Autodesk Fusion 360 part; units mm, degrees
(part 2 of 2)
  constraint concentric A5 A228
  constraint concentric A26 A229
  constraint concentric A24 A230
  constraint concentric A23 A231
  constraint concentric A22 A232
  constraint concentric A21 A233
  constraint concentric A20 A234
  constraint concentric A19 A235
  constraint concentric A18 A236
  constraint concentric A17 A237
  constraint concentric A16 A238
  constraint concentric A15 A239
  constraint concentric A14 A240
  constraint concentric A13 A241
  constraint tangent L211 A241
  constraint tangent A220 L212
  constraint tangent A222 L214
  constraint tangent A240 L232
  constraint tangent A235 L227
  constraint tangent A221 L213
  constraint tangent L212 A221
  constraint tangent A236 L228
  constraint tangent A223 L215
  constraint tangent A224 L216
  constraint tangent A225 L217
  constraint tangent A226 L218
  constraint tangent A239 L231
  constraint tangent A227 L219
  constraint tangent A231 L223
  constraint tangent L219 A228
  constraint tangent A229 L221
  constraint tangent L221 A230
  constraint tangent A234 L226
  constraint tangent A230 L222
  constraint tangent A232 L224
  constraint tangent A233 L225
  constraint tangent A237 L229
  constraint tangent A238 L230
  constraint concentric A220 A242
  constraint concentric A222 A243
  constraint concentric A224 A244
  constraint concentric A225 A245
  constraint concentric A227 A246
  constraint concentric A229 A247
  constraint concentric A230 A248
  constraint concentric A231 A249
  constraint concentric A233 A250
  constraint concentric A235 A251
  constraint concentric A238 A252
  constraint concentric A239 A253
  constraint concentric A240 A254
  constraint tangent A243 L234
  constraint tangent A245 L237
  constraint tangent A246 L239
  constraint tangent A247 L241
  constraint tangent L241 A248
  constraint tangent A253 L248
  constraint tangent A249 L243
  constraint tangent A250 L245
  constraint tangent A254 L249
  constraint tangent A252 L247
  constraint tangent A242 L250
  constraint tangent A243 L251
  constraint tangent A252 L252
  constraint coincident L220 L177.start
  constraint coincident L240 L177.end
  constraint coincident L221 L178.start
  constraint coincident L241 L178.end
  constraint tangent L252 A255
  constraint tangent A255 L253
  constraint tangent A251 L254
  constraint tangent L253 A256
  constraint tangent L254 A256
  constraint tangent L245 A257
  constraint tangent L246 A257
  constraint tangent L243 A258
  constraint tangent L244 A258
  constraint tangent L239 A259
  constraint tangent L240 A259
  constraint tangent L237 A260
  constraint tangent L238 A260
  constraint tangent L234 A261
  constraint tangent L235 A261
  constraint tangent L250 A262
  constraint tangent L251 A262
  constraint tangent L233 A263
  constraint tangent L249 A263
  constraint tangent L203 A264
  constraint tangent L203 A265
  constraint tangent L255 A266
  constraint tangent L255 A267
  measures "d1" diameter of A0
  measures "d2" diameter of A1
  measures "d3" diameter of A2
  measures "d4" diameter of A3
  measures "d5" diameter of A4
  measures "d9" diameter of A111
  measures "d12" diameter of A112
  measures "d396" diameter of A218
  measures "d397" diameter of A219
  measures "d418" radius of A255
  measures "d419" radius of A256
  measures "d420" radius of A257
  measures "d421" radius of A258
  measures "d422" radius of A259
  measures "d423" radius of A260
  measures "d424" radius of A261
  measures "d425" radius of A262
  measures "d426" radius of A263
extrude "Extrude1" add sketch "mriya-bumper-fdm" along normal blind 10.7 contours L177 L178 L211 A220 L212 A221 L213 A222 L214 A223 L215 A224 L216 A225 L217 A226 L218 A227 L219 A228 L220 L221 A230 L222 A231 L223 A232 L224 A233 L225 A234 L226 A235 L227 A236 L228 A237 L229 A238 L230 A239 L231 A240 L232 A241 L233 A242 A243 L234 L235 A244 L236 A245 L237 L238 A246 L239 L240 L241 A248 L242 A249 L243 L244 A250 L245 L246 A251 A252 L247 A253 L248 A254 L249 L250 L251 L252 A255 L253 L254 A256 A257 A258 A259 A260 A261 A262 A263 makes body 1
extrude "Extrude2" add sketch "mriya-bumper-fdm" along normal blind 17.3 contours L177 L178 L220 A229 L221 L240 A247 L241 bodies 1
extrude "Extrude3" add sketch "mriya-bumper-fdm" along normal blind 2 from surface at 1.9 contours A114 | A115 | A116 | A117 | L203 L211 A220 L212 A221 L213 A222 L214 A223 L215 A224 L216 A225 L217 A226 L218 A227 L219 A228 L220 A229 L221 A230 L222 A231 L223 A232 L224 A233 L225 A234 L226 A235 L227 A236 L228 A237 L229 A238 L230 A239 L231 A240 L232 A241 L255 A264 A265 A266 A267 | L203 L220 A264 A265 | L221 L255 A266 A267 bodies 1
extrude "Extrude6" add sketch "mriya-bumper-fdm" along normal blind 1.2 from surface at 14.3 contours L203 L220 A264 A265 bodies 1
extrude "Extrude12" add sketch "mriya-bumper-fdm" along normal blind 1.2 from surface at 7.7 contours L221 L255 A266 A267 bodies 1
sketch "power-switch" plane through (-4.28, 0, 0) normal (1, 0, 0) x (0, 1, 0)
  line L0 (25.7932, 5.6) -> (25.7932, 8.5)
  line L1 (35.9932, 5.6) -> (25.7932, 5.6)
  arc A0 (37.3932, 4.25) -> (37.7932, 4.65) centre (37.3932, 4.65) ccw
  arc A1 (24.3932, 9.85) -> (23.9932, 9.45) centre (24.3932, 9.45) ccw
  line L2 (23.9932, 4.65) -> (23.9932, 9.45)
  line L3 (25.7932, 8.5) -> (35.9932, 8.5)
  arc A2 (23.9932, 4.65) -> (24.3932, 4.25) centre (24.3932, 4.65) ccw
  line L4 (37.7932, 9.45) -> (37.7932, 4.65)
  line L5 (37.3932, 4.25) -> (24.3932, 4.25)
  line L6 (24.3932, 9.85) -> (37.3932, 9.85)
  line L7 (35.9932, 8.5) -> (35.9932, 5.6)
  arc A3 (37.7932, 9.45) -> (37.3932, 9.85) centre (37.3932, 9.45) ccw
  line L8 (1.9932, 0) -> (76.4932, 0)
  line L9 (76.4932, 0) -> (76.4932, 17.3)
  line L10 (76.4932, 17.3) -> (19.3932, 17.3)
  line L11 (19.3932, 17.3) -> (19.3932, 10.7)
  line L12 (19.3932, 10.7) -> (1.9932, 10.7)
  line L13 (1.9932, 10.7) -> (1.9932, 0)
  constraint perpendicular L0 L1
  constraint vertical L0
  constraint perpendicular L0 L3
  constraint vertical L7
  constraint tangent L6 A3
  constraint tangent L4 A3
  constraint tangent A0 L4
  constraint tangent A0 L5
  constraint tangent A2 L5
  constraint tangent L2 A2
  constraint tangent A1 L2
  constraint tangent A1 L6
extrude "Extrude8" cut sketch "power-switch" against normal blind 2.6 contours L0 L1 L3 L7 bodies 1
extrude "Extrude9" cut sketch "power-switch" against normal blind 1.2 contours A0 A1 L2 A2 L4 L5 L6 A3 bodies 1
chamfer "Chamfer13" distance 1.43 angle 40 8 edges at (-4.28, 30.8932, 4.25) (-4.28, 24.1104, 4.3672) (-4.28, 23.9932, 7.05) (-4.28, 24.1104, 9.7328) (-4.28, 30.8932, 9.85) (-4.28, 37.676, 9.7328) (-4.28, 37.7932, 7.05) (-4.28, 37.676, 4.3672) measured on face at (-4.28, 63.5932, 8.9167) measured on face at (-4.28, 63.5932, 8.9167) measured on face at (-4.28, 63.5932, 8.9167) measured on face at (-4.28, 63.5932, 8.9167) measured on face at (-4.28, 63.5932, 8.9167) measured on face at (-4.28, 63.5932, 8.9167) measured on face at (-4.28, 63.5932, 8.9167) measured on face at (-4.28, 63.5932, 8.9167) on bodies 1
sketch "usb-c" plane through (0, 80.8132, 0) normal (0, 1, 0) x (-1, 0, 0)
  line L0 (11.0002, 8.4) -> (11.0002, 13.2)
  line L1 (21.0002, 11.4) -> (21.0002, 10.2)
  line L2 (11.8003, 10.2) -> (11.8003, 11.4)
  arc A0 (11.4002, 13.6) -> (11.0002, 13.2) centre (11.4002, 13.2) ccw
  line L3 (11.4002, 13.6) -> (21.4002, 13.6)
  line L4 (21.8003, 13.2) -> (21.8003, 8.4)
  arc A1 (21.8003, 13.2) -> (21.4002, 13.6) centre (21.4002, 13.2) ccw
  arc A2 (21.4002, 8) -> (21.8002, 8.4) centre (21.4002, 8.4) ccw
  line L5 (13.0003, 12.6) -> (19.8002, 12.6)
  line L6 (19.8002, 9) -> (13.0003, 9)
  line L7 (21.4002, 8) -> (11.4002, 8)
  arc A3 (11.0002, 8.4) -> (11.4002, 8) centre (11.4002, 8.4) ccw
  arc A4 (21.0002, 11.4) -> (19.8002, 12.6) centre (19.8002, 11.4) ccw
  arc A5 (19.8002, 9) -> (21.0002, 10.2) centre (19.8002, 10.2) ccw
  arc A6 (13.0003, 12.6) -> (11.8003, 11.4) centre (13.0003, 11.4) ccw
  arc A7 (11.8003, 10.2) -> (13.0003, 9) centre (13.0003, 10.2) ccw
  line L8 (8.6, 0) -> (41.0177, 0)
  line L9 (41.0177, 0) -> (41.0177, 10.7)
  line L10 (41.0177, 10.7) -> (25.7, 10.7)
  line L11 (25.7, 10.7) -> (25.7, 17.3)
  line L12 (25.7, 17.3) -> (8.6, 17.3)
  line L13 (8.6, 17.3) -> (8.6, 0)
  constraint perpendicular L3 L4
  constraint perpendicular L0 L7
  constraint horizontal L7
  constraint perpendicular L4 L7
  constraint tangent A0 L3
  constraint tangent L0 A0
  constraint tangent L3 A1
  constraint tangent L4 A1
  constraint tangent L0 A3
  constraint tangent L7 A3
  constraint tangent A2 L7
  constraint tangent L4 A2
  constraint tangent L5 A4
  constraint tangent L1 A4
  constraint tangent L1 A5
  constraint tangent L6 A5
  constraint tangent L2 A6
  constraint tangent L5 A6
  constraint tangent L6 A7
  constraint tangent L2 A7
extrude "Extrude13" cut sketch "usb-c" against normal blind 2.6 contours L1 L2 L5 L6 A4 A5 A6 A7 bodies 1
extrude "Extrude15" cut sketch "usb-c" against normal blind 1.2 contours L0 A0 L3 L4 A1 A2 L7 A3 bodies 1
chamfer "Chamfer31" distance 1.2 angle 45 8 edges at (-16.4003, 80.8132, 8) (-11.1174, 80.8132, 8.1172) (-11.0003, 80.8132, 10.8) (-11.1174, 80.8132, 13.4828) (-16.4003, 80.8132, 13.6) (-21.6831, 80.8132, 13.4828) (-21.8003, 80.8132, 10.8) (-21.6831, 80.8132, 8.1172) on bodies 1
chamfer "Chamfer27" distance 1 angle 45 43 edges at (-4.28, 10.6932, 10.7) (-33.3589, 80.8132, 10.7) (-41.4004, 80.8893, 10.7) (-42.0225, 81.4038, 10.7) (-43.8839, 82.7463, 10.7) (-51.773, 83.1132, 10.7) (-58.2004, 83.1893, 10.7) (-59.9225, 84.8038, 10.7) (-62.8839, 87.2463, 10.7) (-73.4, 87.6132, 10.7) (-83.9161, 87.2463, 10.7) (-86.3775, 85.3038, 10.7) (-87.5996, 84.1893, 10.7) (-94.5269, 84.1132, 10.7) (-102.9161, 83.7463, 10.7) (-107.4811, 79.7002, 10.7) (-111.1311, 76.2654, 10.7) (-115.9841, 76.1132, 10.7) (-121.9161, 75.7463, 10.7) (-123.7775, 74.4038, 10.7) (-124.3996, 73.8893, 10.7) (-131.4411, 73.8132, 10.7) (-141.1547, 72.5479, 10.7) (-142.42, 42.8932, 10.7) (-141.1547, 13.2385, 10.7) (-120.6213, 11.9732, 10.7) (-100.9154, 12.4162, 10.7) (-96.1725, 16.5326, 10.7) (-92.6689, 19.821, 10.7) (-84.6, 19.9732, 10.7) (-75.7843, 19.5642, 10.7) (-70.8069, 11.5856, 10.7) (-65.1622, 2.9302, 10.7) (-55.7575, 2.2732, 10.7) (-48.3996, 2.1971, 10.7) (-47.7775, 1.6826, 10.7) (-45.9161, 0.3401, 10.7) (-36.927, -0.0268, 10.7) (-29.3996, -0.1029, 10.7) (-28.7775, -0.6174, 10.7) (-26.9161, -1.9599, 10.7) (-16.8358, -2.3268, 10.7) (-5.5453, -1.0615, 10.7) measured on face at (-140.6867, 34.0265, 10.7) measured on face at (-140.6867, 34.0265, 10.7) measured on face at (-140.6867, 34.0265, 10.7) measured on face at (-140.6867, 34.0265, 10.7) measured on face at (-140.6867, 34.0265, 10.7) measured on face at (-140.6867, 34.0265, 10.7) measured on face at (-140.6867, 34.0265, 10.7) measured on face at (-140.6867, 34.0265, 10.7) measured on face at (-140.6867, 34.0265, 10.7) measured on face at (-140.6867, 34.0265, 10.7) measured on face at (-140.6867, 34.0265, 10.7) measured on face at (-140.6867, 34.0265, 10.7) measured on face at (-140.6867, 34.0265, 10.7) measured on face at (-140.6867, 34.0265, 10.7) measured on face at (-140.6867, 34.0265, 10.7) measured on face at (-140.6867, 34.0265, 10.7) measured on face at (-140.6867, 34.0265, 10.7) measured on face at (-140.6867, 34.0265, 10.7) measured on face at (-140.6867, 34.0265, 10.7) measured on face at (-140.6867, 34.0265, 10.7) measured on face at (-140.6867, 34.0265, 10.7) measured on face at (-140.6867, 34.0265, 10.7) measured on face at (-140.6867, 34.0265, 10.7) measured on face at (-140.6867, 34.0265, 10.7) measured on face at (-140.6867, 34.0265, 10.7) measured on face at (-140.6867, 34.0265, 10.7) measured on face at (-140.6867, 34.0265, 10.7) measured on face at (-140.6867, 34.0265, 10.7) measured on face at (-140.6867, 34.0265, 10.7) measured on face at (-140.6867, 34.0265, 10.7) measured on face at (-140.6867, 34.0265, 10.7) measured on face at (-140.6867, 34.0265, 10.7) measured on face at (-140.6867, 34.0265, 10.7) measured on face at (-140.6867, 34.0265, 10.7) measured on face at (-140.6867, 34.0265, 10.7) measured on face at (-140.6867, 34.0265, 10.7) measured on face at (-140.6867, 34.0265, 10.7) measured on face at (-140.6867, 34.0265, 10.7) measured on face at (-140.6867, 34.0265, 10.7) measured on face at (-140.6867, 34.0265, 10.7) measured on face at (-140.6867, 34.0265, 10.7) measured on face at (-140.6867, 34.0265, 10.7) measured on face at (-140.6867, 34.0265, 10.7) on bodies 1
chamfer "Chamfer28" distance 1 angle 45 44 edges at (-4.28, 39.2432, 0) (-5.5453, 79.5479, 0) (-24.8089, 80.8132, 0) (-41.4004, 80.8893, 0) (-42.0225, 81.4038, 0) (-43.8839, 82.7463, 0) (-51.773, 83.1132, 0) (-58.2004, 83.1893, 0) (-59.9225, 84.8038, 0) (-62.8839, 87.2463, 0) (-73.4, 87.6132, 0) (-83.9161, 87.2463, 0) (-86.3775, 85.3038, 0) (-87.5996, 84.1893, 0) (-94.5269, 84.1132, 0) (-102.9161, 83.7463, 0) (-107.4811, 79.7002, 0) (-111.1311, 76.2654, 0) (-115.9841, 76.1132, 0) (-121.9161, 75.7463, 0) (-123.7775, 74.4038, 0) (-124.3996, 73.8893, 0) (-131.4411, 73.8132, 0) (-141.1547, 72.5479, 0) (-142.42, 42.8932, 0) (-141.1547, 13.2385, 0) (-120.6213, 11.9732, 0) (-100.9154, 12.4162, 0) (-96.1725, 16.5326, 0) (-92.6689, 19.821, 0) (-84.6, 19.9732, 0) (-75.7843, 19.5642, 0) (-70.8069, 11.5856, 0) (-65.1622, 2.9302, 0) (-55.7575, 2.2732, 0) (-48.3996, 2.1971, 0) (-47.7775, 1.6826, 0) (-45.9161, 0.3401, 0) (-36.927, -0.0268, 0) (-29.3996, -0.1029, 0) (-28.7775, -0.6174, 0) (-26.9161, -1.9599, 0) (-16.8358, -2.3268, 0) (-5.5453, -1.0615, 0) measured on face at (-4.28, 64.0698, 8.9167) measured on face at (-4.7602, 78.4727, 11.5333) measured on face at (-6.0133, 51.6599, 0) measured on face at (-6.0133, 51.6599, 0) measured on face at (-41.9233, 81.3045, 3.2333) measured on face at (-42.6302, 81.9855, 6.4667) measured on face at (-6.0133, 51.6599, 0) measured on face at (-6.0133, 51.6599, 0) measured on face at (-6.0133, 51.6599, 0) measured on face at (-62.6914, 87.1616, 6.4667) measured on face at (-6.0133, 51.6599, 0) measured on face at (-84.1086, 87.1616, 6.4667) measured on face at (-86.0783, 85.603, 3.2333) measured on face at (-6.0133, 51.6599, 0) measured on face at (-6.0133, 51.6599, 0) measured on face at (-103.1086, 83.6616, 6.4667) measured on face at (-6.0133, 51.6599, 0) measured on face at (-6.0133, 51.6599, 0) measured on face at (-6.0133, 51.6599, 0) measured on face at (-121.1148, 75.9989, 6.4667) measured on face at (-6.0133, 51.6599, 0) measured on face at (-6.0133, 51.6599, 0) measured on face at (-6.0133, 51.6599, 0) measured on face at (-142.3419, 70.3108, 6.4667) measured on face at (-142.42, 51.7599, 3.2333) measured on face at (-140.6058, 12.7742, 6.4667) measured on face at (-114.7951, 11.9732, 6.4667) measured on face at (-102.6354, 11.9953, 3.2333) measured on face at (-6.0133, 51.6599, 0) measured on face at (-6.0133, 51.6599, 0) measured on face at (-87.0345, 19.9732, 3.2333) measured on face at (-6.0133, 51.6599, 0) measured on face at (-6.0133, 51.6599, 0) measured on face at (-66.4491, 4.0238, 6.4667) measured on face at (-6.0133, 51.6599, 0) measured on face at (-6.0133, 51.6599, 0) measured on face at (-6.0133, 51.6599, 0) measured on face at (-47.3279, 1.2395, 3.2333) measured on face at (-34.5454, -0.0268, 6.4667) measured on face at (-6.0133, 51.6599, 0) measured on face at (-6.0133, 51.6599, 0) measured on face at (-27.6614, -1.5719, 6.4667) measured on face at (-6.0133, 51.6599, 0) measured on face at (-5.081, -0.5126, 6.4667) on bodies 1
fillet "Fillet30" radius 1.2 2 edges at (-4.28, 19.3932, 13.5) (-25.7, 80.8132, 13.5) on bodies 1
chamfer "Chamfer29" distance 1 angle 45 7 edges at (-4.28, 48.5432, 17.3) (-5.5453, 79.5479, 17.3) (-16.55, 80.8132, 17.3) (-25.3485, 80.4617, 17.3) (-25.7, 78.9132, 17.3) (-6.18, 19.3932, 17.3) (-4.6315, 19.7447, 17.3) measured on face at (-6.0133, 38.8265, 17.3) measured on face at (-6.0133, 38.8265, 17.3) measured on face at (-6.0133, 38.8265, 17.3) measured on face at (-24.5991, 80.8091, 14.7689) measured on face at (-6.0133, 38.8265, 17.3) measured on face at (-6.0133, 38.8265, 17.3) measured on face at (-4.2841, 20.4941, 14.7689) on bodies 1
chamfer "Chamfer34" distance 0.7 angle 45 2 edges at (-6.88, 9.5932, 7.7) (-16.4, 78.2132, 14.3) on bodies 1
mirror "Mirror1" about plane through (0, 0, 0) normal (1, 0, 0) of bodies 1 makes body 2
named bodies: "Left", "Right"
